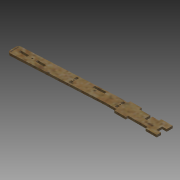
# Autodesk Inventor part: ArmInsideLow
Saved by Autodesk Inventor 2012 (Build 160160000, 160)
## iProperties
Created: 2014-07-02
Part Number: ArmInsideLow
Material: Default
Document SubType Name: Modeling
Designer: Laurent
Density: 1 g/cm^3
RuleStatus: InUse
Author: Laurent
Autodesk Inventor part; units mm, degrees
ref_plane "YZ Plane" through (0, 0, 0) normal (1, 0, 0) x (0, 1, 0)
ref_plane "XZ Plane" through (0, 0, 0) normal (0, 1, 0) x (-1, 0, 0)
ref_plane "XY Plane" through (0, 0, 0) normal (0, 0, 1) x (1, 0, 0)
sketch "Sketch1" plane through (0, 0, 0) normal (0, 0, 1) x (1, 0, 0)
  line L0 (-130, 16.5) -> (130, 16.5)
  line L1 (130, 16.5) -> (130, -16.5)
  line L2 (130, -16.5) -> (-130, -16.5)
  line L3 (-130, -16.5) -> (-130, 16.5)
  point P0 (0, 0)
  dimension "d0" = 260
  dimension "d1" = 33
  dimension "d2" = 16.5
  dimension "d3" = 130
  constraints: 8 end point, 2 parallel, 1 horizontal, 1 perpendicular
  measures "d0" distance of L1.end L2.end
  measures "d1" distance of L0.end L1.end
  measures "d2" distance from line of L2 point (0, 0)
  measures "d3" distance from line of L3 point (0, 0)
extrude "Base" add sketch "Sketch1" along normal blind 4
sketch "Sketch2" plane through (0, 0, 4) normal (0, 0, 1) x (1, 0, 0)
  line L0 (130, 16.5) -> (130, -16.5) projected
  line L1 (-130, 16.5) -> (130, 16.5) projected
  line L2 (-130, -16.5) -> (-130, 16.5) projected
  line L3 (130, -16.5) -> (-130, -16.5) projected
  line L4 (75, 16.5) -> (110, 16.5)
  line L5 (110, 16.5) -> (110, 12.5)
  line L6 (110, 12.5) -> (75, 12.5)
  line L7 (75, 12.5) -> (75, 16.5)
  line L8 (-130, 16.5) -> (55, 16.5)
  line L9 (55, 16.5) -> (55, 12.5)
  line L10 (55, 12.5) -> (-130, 12.5)
  line L11 (-130, 12.5) -> (-130, 16.5)
  line L12 (35, -7.5) -> (55, -7.5)
  line L13 (55, -7.5) -> (55, -16.5)
  line L14 (55, -16.5) -> (35, -16.5)
  line L15 (35, -16.5) -> (35, -7.5)
  line L16 (75, -7.5) -> (110, -7.5)
  line L17 (110, -7.5) -> (110, -16.5)
  line L18 (110, -16.5) -> (75, -16.5)
  line L19 (75, -16.5) -> (75, -7.5)
  line L20 (110, -11.5) -> (130, -11.5)
  line L21 (130, -11.5) -> (130, -16.5)
  line L22 (130, -16.5) -> (110, -16.5)
  line L23 (110, -16.5) -> (110, -11.5)
  line L24 (55, -11.5) -> (75, -11.5)
  line L25 (75, -11.5) -> (75, -16.5)
  line L26 (75, -16.5) -> (55, -16.5)
  line L27 (55, -16.5) -> (55, -11.5)
  point P0 (0, 0)
  dimension "d6" = 35
  dimension "d7" = 4
  dimension "d8" = 0
  dimension "d9" = 20
  dimension "d10" = 185
  dimension "d11" = 4
  dimension "d12" = 0
  dimension "d13" = 0
  dimension "d14" = 20
  dimension "d15" = 20
  dimension "d16" = 9
  dimension "d17" = 0
  dimension "d18" = 165
  dimension "d19" = 35
  dimension "d20" = 9
  dimension "d21" = 0
  dimension "d22" = 20
  dimension "d23" = 20
  dimension "d24" = 5
  dimension "d25" = 20
  dimension "d26" = 5
  dimension "d27" = 0
  dimension "d28" = 0
  dimension "d29" = 0
  dimension "d30" = 0
  dimension "d98" = 20
  constraints: 48 end point, 12 parallel, 6 horizontal, 6 perpendicular
  measures "d6" distance of L5.end L6.end
  measures "d7" distance of L4.end L5.end
  measures "d8" distance between parallel lines of L1 L4
  measures "d9" distance from line of L0 L5.end
  measures "d10" distance of L9.end L10.end
  measures "d11" distance of L8.end L9.end
  measures "d12" distance between parallel lines of L2 L11
  measures "d13" distance between parallel lines of L1 L8
  measures "d14" distance between parallel lines of L7 L9
  measures "d15" distance of L13.end L14.end
  measures "d16" distance of L12.end L13.end
  measures "d17" distance between parallel lines of L3 L14
  measures "d18" distance between parallel lines of L2 L15
  measures "d19" distance of L17.end L18.end
  measures "d20" distance of L16.end L17.end
  measures "d21" distance between parallel lines of L3 L18
  measures "d22" distance between parallel lines of L0 L17
  measures "d23" distance of L21.end L22.end
  measures "d24" distance of L20.end L21.end
  measures "d25" distance of L25.end L26.end
  measures "d26" distance of L24.end L25.end
  measures "d27" distance between parallel lines of L3 L22
  measures "d28" distance between parallel lines of L0 L21
  measures "d29" distance between parallel lines of L3 L26
  measures "d30" distance between parallel lines of L13 L27
  measures "d98" distance between parallel lines of L16 L6
extrude "StructureMounting" cut sketch "Sketch2" against normal blind 4 contours L0 L3 L17 L20 | L5 L6 L7 L1 | L17 L3 L19 L16 | L9 L10 L2 L1 | L3 L13 L24 L19 | L3 L15 L12 L13
sketch "Sketch4" plane through (0, 0, 4) normal (0, 0, 1) x (1, 0, 0)
  line L0 (55, 12.5) -> (-130, 12.5) projected
  line L1 (-130, -16.5) -> (-130, 12.5) projected
  line L2 (35, -16.5) -> (-130, -16.5) projected
  line L3 (35, -16.5) -> (35, -7.5) projected
  line L4 (55, 16.5) -> (55, 12.5) projected
  line L5 (35, -7.5) -> (-130, -16.5)
  line L6 (-130, 3.5) -> (35, 12.5)
  point P0 (0, 0)
  dimension "d42" = 20
  dimension "d43" = 20
  constraints: 4 end point, 4 point on line
  measures "d42" distance from line of L2 L6.start
  measures "d43" distance from line of L4 L6.end
extrude "MotorRamp" cut sketch "Sketch4" against normal blind 4
sketch "Sketch5" plane through (0, 0, 4) normal (0, 0, 1) x (1, 0, 0)
  line L0 (110, 12.5) -> (75, 12.5) projected
  line L1 (75, 12.5) -> (75, 16.5) projected
  line L2 (94.274, 12.5) -> (98.274, 12.5)
  line L3 (98.274, 12.5) -> (98.274, 2.5)
  line L4 (98.274, 2.5) -> (94.274, 2.5)
  line L5 (94.274, 2.5) -> (94.274, 12.5)
  line L6 (110, 16.5) -> (110, 12.5) projected
  point P0 (0, 0)
  dimension "d46" = 4
  dimension "d47" = 10
  dimension "d48" = 0
  dimension "d49" = 19.274
  dimension "d100" = 11.726
  constraints: 8 end point, 2 parallel, 1 horizontal, 1 perpendicular
  measures "d46" distance of L3.end L4.end
  measures "d47" distance of L2.end L3.end
  measures "d48" distance between parallel lines of L0 L2
  measures "d49" distance between parallel lines of L1 L5
  measures "d100" distance between parallel lines of L6 L3
extrude "LowSleeve" cut sketch "Sketch5" against normal blind 4
sketch "Sketch6" plane through (0, 0, 4) normal (0, 0, 1) x (1, 0, 0)
  line L0 (-130, -16.5) -> (-130, 3.5) projected
  line L1 (-120, -2.5) -> (-105, -2.5)
  line L2 (-105, -2.5) -> (-105, -6.5)
  line L3 (-105, -6.5) -> (-120, -6.5)
  line L4 (-120, -6.5) -> (-120, -2.5)
  line L5 (-90, -2.5) -> (-75, -2.5)
  line L6 (-75, -2.5) -> (-75, -6.5)
  line L7 (-75, -6.5) -> (-90, -6.5)
  line L8 (-90, -6.5) -> (-90, -2.5)
  line L9 (98.274, 2.5) -> (94.274, 2.5) projected
  line L10 (-106.4171, -4.5) -> (-87.4505, -4.5) construction
  circle A0 centre (-97.5, -4.5) radius 1.25
  point P0 (0, 0)
  dimension "d63" = 15
  dimension "d64" = 4
  dimension "d67" = 30
  dimension "d72" = 10
  dimension "d73" = 10
  dimension "d166" = 2
  dimension "d167" = 2.5
  dimension "d168" = 7.5
  constraints: 18 end point, 3 parallel, 2 horizontal, 1 centre point, 1 collinear, 1 perpendicular, 1 point on line, 7 other
  measures "d63" distance of L2.end L3.end
  measures "d64" distance of L1.end L2.end
  measures "d67" distance of L1.start L8.end
  measures "d72" distance from line of L0.start L3
  measures "d73" distance between parallel lines of L0 L4
  measures "d166" distance between parallel lines of L10 L1
  measures "d167" diameter of A0
  measures "d168" distance from line of L2 A0.centre
extrude "MotorSleeves" cut sketch "Sketch6" against normal blind 4
sketch "Sketch10" plane through (0, 0, 4) normal (0, 0, 1) x (1, 0, 0)
  line L0 (130, 16.5) -> (130, -11.5) projected
  line L1 (122, 6) -> (130, 6)
  line L2 (130, 6) -> (130, -4)
  line L3 (130, -4) -> (122, -4)
  line L4 (122, -4) -> (122, 6)
  point P0 (0, 0)
  dimension "d109" = 8
  dimension "d110" = 10
  dimension "d111" = 0
  dimension "d112" = 4
  constraints: 8 end point, 2 parallel, 1 horizontal, 1 perpendicular
  measures "d109" distance of L2.end L3.end
  measures "d110" distance between parallel lines of L1 L3
  measures "d111" distance between parallel lines of L0 L2
  measures "d112" distance from line of point (0, 0) L3
extrude "Cabling" cut sketch "Sketch10" against normal blind 4
sketch "Sketch12" plane through (0, 0, 4) normal (0, 0, 1) x (1, 0, 0)
  line L0 (35, 12.5) -> (-130, 3.5) projected
  line L1 (-0.084, 8.5834) -> (19.8863, 9.6726)
  line L2 (19.8863, 9.6726) -> (20.1041, 5.6786)
  line L3 (20.1041, 5.6786) -> (0.1338, 4.5893)
  line L4 (0.1338, 4.5893) -> (-0.084, 8.5834)
  point P0 (0, 0)
  dimension "d124" = 4
  dimension "d125" = 20
  dimension "d126" = 2
  dimension "d127" = 130
  constraints: 8 end point, 2 parallel, 1 perpendicular
  measures "d124" distance of L1.end L2.end
  measures "d125" distance between parallel lines of L2 L4
  measures "d126" distance between parallel lines of L0 L1
  measures "d127" distance from line of L4 L0.end
extrude "ESCholder" cut sketch "Sketch12" against normal blind 4
sketch "Sketch13" plane through (0, 0, 4) normal (0, 0, 1) x (1, 0, 0)
  line L0 (55, 16.5) -> (55, 12.5) projected
  line L1 (55, 12.5) -> (35, 12.5) projected
  line L2 (35, 12.5) -> (-130, 3.5) projected
  line L3 (-130, -16.5) -> (35, -7.5) projected
  line L4 (-30.0123, 6.4502) -> (-26.0182, 6.668)
  line L5 (-26.0182, 6.668) -> (-25.7459, 1.6754)
  line L6 (-25.7459, 1.6754) -> (-29.7399, 1.4576)
  line L7 (-29.7399, 1.4576) -> (-30.0123, 6.4502)
  line L8 (-47.5366, -2.0169) -> (-6.9954, 0.1945) construction
  line L9 (-29.1953, -8.5276) -> (-25.2012, -8.3097)
  line L10 (-25.2012, -8.3097) -> (-25.4736, -3.3171)
  line L11 (-25.4736, -3.3171) -> (-29.4676, -3.535)
  line L12 (-29.4676, -3.535) -> (-29.1953, -8.5276)
  line L13 (20.1041, 5.6786) -> (0.1338, 4.5893) projected
  line L14 (-27.9377, 5.1382) -> (-27.2725, -7.0585) construction
  circle A0 centre (-27.6051, -0.9601) radius 1.25
  line L15 (49, 10) -> (53, 10)
  line L16 (53, 10) -> (53, 5)
  line L17 (53, 5) -> (49, 5)
  line L18 (49, 5) -> (49, 10)
  line L19 (39.5253, 2.5) -> (63.8345, 2.5) construction
  line L20 (49, -5) -> (53, -5)
  line L21 (53, -5) -> (53, 0)
  line L22 (53, 0) -> (49, 0)
  line L23 (49, 0) -> (49, -5)
  circle A1 centre (51, 2.5) radius 1.25
  point P0 (0, 0)
  dimension "d134" = 2.5
  dimension "d135" = 7.5
  dimension "d136" = 4
  dimension "d137" = 100
  dimension "d140" = 10
  dimension "d151" = 2
  dimension "d152" = 2.5
  dimension "d153" = 4
  dimension "d154" = 5
  dimension "d155" = 2.5
  dimension "d156" = 6
  dimension "d157" = 10
  dimension "d158" = 2.5
  dimension "d159" = 2
  constraints: 38 end point, 8 parallel, 8 symmetric about line, 5 perpendicular, 2 centre point, 1 coincident, 1 horizontal, 1 midpoint, 1 point on line
  measures "d134" distance between parallel lines of L2 L4
  measures "d135" distance between parallel lines of L2 L6
  measures "d136" distance between parallel lines of L5 L7
  measures "d137" distance from line of L2.end L7
  measures "d140" distance between parallel lines of L2 L8
  measures "d151" distance between parallel lines of L7 L14
  measures "d152" diameter of A0
  measures "d153" distance of L16.end L17.end
  measures "d154" distance of L15.end L16.end
  measures "d155" distance between parallel lines of L1 L15
  measures "d156" distance between parallel lines of L0 L18
  measures "d157" distance between parallel lines of L1 L19
  measures "d158" diameter of A1
  measures "d159" distance from line of L18 A1.centre
extrude "CrossSupports" cut sketch "Sketch13" against normal blind 10
sketch "Sketch14" plane through (0, 0, 4) normal (0, 0, 1) x (1, 0, 0)
  line L0 (110, 12.5) -> (75, 12.5) projected
  circle A0 centre (113, 8) radius 3
  circle A1 centre (105, 8) radius 3
  point P0 (98.274, 12.5)
  point P1 (0, 0)
  dimension "d141" = 6
  dimension "d142" = 6
  dimension "d143" = 4.5
  dimension "d144" = 4.5
  dimension "d145" = 3
  dimension "d146" = 8
  constraints: 2 centre point
  measures "d141" diameter of A0
  measures "d142" diameter of A1
  measures "d143" distance from line of L0 A1.centre
  measures "d144" distance from line of L0 A0.centre
  measures "d145" horizontal distance of L0.start A0.centre
  measures "d146" distance of A0.centre A1.centre
extrude "ESCpowerHoles" [suppressed]
sketch "Sketch15" plane through (0, 0, 4) normal (0, 0, 1) x (1, 0, 0)
  line L0 (75, -7.5) -> (110, -7.5) projected
  line L1 (94.274, 2.5) -> (98.274, 2.5)
  line L2 (98.274, 2.5) -> (98.274, -7.5)
  line L3 (98.274, -7.5) -> (94.274, -7.5)
  line L4 (94.274, -7.5) -> (94.274, 2.5)
  point P0 (0, 0)
  constraints: 8 end point, 2 parallel, 1 horizontal, 1 perpendicular, 1 point on line
extrude "HighSleeve" [suppressed]
sketch "Sketch16" plane through (0, 0, 4) normal (0, 0, 1) x (1, 0, 0)
  line L0 (-130, -16.5) -> (-130, 3.5) projected
  line L1 (-128, 1.5) -> (-126.4, 1.5)
  line L2 (-126.4, 1.5) -> (-126.4, -13.5)
  line L3 (-126.4, -13.5) -> (-128, -13.5)
  line L4 (-128, -13.5) -> (-128, 1.5)
  point P0 (0, 0)
  dimension "d160" = 1.6
  dimension "d161" = 15
  dimension "d162" = 2
  dimension "d163" = 2
  constraints: 8 end point, 2 parallel, 1 horizontal, 1 perpendicular
  measures "d160" distance of L2.end L3.end
  measures "d161" distance of L1.end L2.end
  measures "d162" distance between parallel lines of L0 L4
  measures "d163" distance from line of L0.end L1
extrude "WingLedCutout" cut sketch "Sketch16" against normal blind 10
fillet "ImpactReduction" radius 5 2 edges at (-130, 3.5, 2) (-130, -16.5, 2)
body "Solid1"
